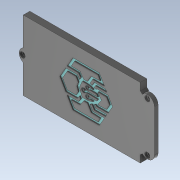
# Autodesk Inventor part: BodyBotSup
Saved by Autodesk Inventor 2020 (Build 240168000, 168)
## iProperties
Created: 2020-02-29
Part Number: BodyBotSup
Material: Generic
Document SubType Name: Modeling
Designer: Turing
Density: 1 g/cm^3
Appearance: Smooth - Black
Mass: 46.7134 g
Surface Area: 265.653 cm^2
Volume: 46.7134 cm^3
Author: Turing
Autodesk Inventor part; units mm, degrees
ref_plane "YZ Plane" through (0, 0, 0) normal (1, 0, 0) x (0, 1, 0)
ref_plane "XZ Plane" through (0, 0, 0) normal (0, 1, 0) x (-1, 0, 0)
ref_plane "XY Plane" through (0, 0, 0) normal (0, 0, 1) x (1, 0, 0)
sketch "Sketch1" plane through (0, 0, 0) normal (0, 0, 1) x (1, 0, 0)
  circle A0 centre (-91.4877, 59.6152) radius 5 projected
  circle A1 centre (0, -76.8001) radius 5 projected
  circle A2 centre (91.4877, 59.6152) radius 5 projected
  circle A3 centre (91.4877, -59.6152) radius 5 projected
  circle A4 centre (-91.4877, -59.6152) radius 5 projected
  circle A5 centre (0, 76.8001) radius 5 projected
  line L0 (-72.1, 6.8739) -> (-72.1, 37.6) projected
  line L1 (-72.1, 37.6) -> (53.9, 37.6) projected
  line L2 (53.9, 37.6) -> (53.9, 29.7386) projected
  line L3 (53.9, 29.7386) -> (56.1, 27.699) projected
  arc A6 (69.1, 22.6) -> (56.1, 27.699) centre (61.6, 22.6) ccw projected
  line L4 (69.1, 22.6) -> (69.1, -22.6) projected
  arc A7 (56.1, -27.699) -> (69.1, -22.6) centre (61.6, -22.6) ccw projected
  line L5 (56.1, -27.699) -> (53.9, -29.7386) projected
  line L6 (53.9, -29.7386) -> (53.9, -37.6) projected
  line L7 (53.9, -37.6) -> (-72.1, -37.6) projected
  line L8 (-72.1, -37.6) -> (-72.1, -6.8739) projected
  arc A8 (-72.1, 6.8739) -> (-72.1, -6.8739) centre (-69.1, 0) ccw projected
  line L9 (53.9, 29.7386) -> (56.1, 27.699) projected
  line L10 (53.9, 37.6) -> (53.9, 29.7386) projected
  line L11 (-72.1, 37.6) -> (53.9, 37.6) projected
  line L12 (-72.1, 6.8739) -> (-72.1, 37.6) projected
  arc A9 (-69.1, 7.5) -> (-72.1, 6.8739) centre (-69.1, 0) ccw projected
  line L13 (-69.1, 34.6) -> (-69.1, 7.5) projected
  line L14 (50.9, 34.6) -> (-69.1, 34.6) projected
  line L15 (50.9, 26.6) -> (50.9, 34.6) projected
  line L16 (-60, 26.6) -> (50.9, 26.6) projected
  line L17 (-60, 22.6) -> (-60, 26.6) projected
  line L18 (54.1, 22.6) -> (-60, 22.6) projected
  arc A10 (56.1, 27.699) -> (54.1, 22.6) centre (61.6, 22.6) ccw projected
  line L19 (53.9, -37.6) -> (-72.1, -37.6) projected
  line L20 (53.9, -29.7386) -> (53.9, -37.6) projected
  line L21 (56.1, -27.699) -> (53.9, -29.7386) projected
  arc A11 (54.1, -22.6) -> (56.1, -27.699) centre (61.6, -22.6) ccw projected
  line L22 (-60, -22.6) -> (54.1, -22.6) projected
  line L23 (-60, -26.6) -> (-60, -22.6) projected
  line L24 (50.9, -26.6) -> (-60, -26.6) projected
  line L25 (50.9, -34.6) -> (50.9, -26.6) projected
  line L26 (-69.1, -34.6) -> (50.9, -34.6) projected
  line L27 (-69.1, -7.5) -> (-69.1, -34.6) projected
  arc A12 (-72.1, -6.8739) -> (-69.1, -7.5) centre (-69.1, 0) ccw projected
  line L28 (-72.1, -37.6) -> (-72.1, -6.8739) projected
  circle A13 centre (-72.85, 0) radius 1.5 projected
  circle A14 centre (61.6, -26.35) radius 1.5 projected
  circle A15 centre (61.6, 26.35) radius 1.5 projected
  line L29 (-77.315, -35.1795) -> (-80.415, -33.3898) projected
  line L30 (-80.415, -33.3898) -> (-80.415, -29.8103) projected
  line L31 (-80.415, -29.8103) -> (-77.315, -28.0205) projected
  line L32 (-77.315, -28.0205) -> (-74.2151, -29.8102) projected
  line L33 (-74.2151, -29.8102) -> (-74.2151, -33.3897) projected
  line L34 (-74.2151, -33.3897) -> (-77.315, -35.1795) projected
  line L35 (-1.7898, 50.8) -> (1.7897, 50.8) projected
  line L36 (1.7897, 50.8) -> (3.5795, 47.7) projected
  line L37 (3.5795, 47.7) -> (1.7897, 44.6001) projected
  line L38 (1.7897, 44.6001) -> (-1.7898, 44.6001) projected
  line L39 (-1.7898, 44.6001) -> (-3.5795, 47.7) projected
  line L40 (-3.5795, 47.7) -> (-1.7898, 50.8) projected
  line L41 (-74.2151, 33.3898) -> (-74.2151, 29.8103) projected
  line L42 (-74.2151, 29.8103) -> (-77.315, 28.0205) projected
  line L43 (-77.315, 28.0205) -> (-80.415, 29.8102) projected
  line L44 (-80.415, 29.8102) -> (-80.415, 33.3897) projected
  line L45 (-80.415, 33.3897) -> (-77.315, 35.1795) projected
  line L46 (-77.315, 35.1795) -> (-74.2151, 33.3898) projected
  line L47 (1.7897, -50.8) -> (-1.7898, -50.8) projected
  line L48 (-1.7898, -50.8) -> (-3.5795, -47.7) projected
  line L49 (-3.5795, -47.7) -> (-1.7898, -44.6001) projected
  line L50 (-1.7898, -44.6001) -> (1.7897, -44.6001) projected
  line L51 (1.7897, -44.6001) -> (3.5795, -47.7) projected
  line L52 (3.5795, -47.7) -> (1.7897, -50.8) projected
  line L53 (94.3529, -43.81) -> (76.3482, 0) projected
  line L54 (76.3482, 0) -> (94.3529, 43.81) projected
  arc A16 (13.202, 67.65) -> (75.5922, 62.4195) centre (47.6542, 103.886) ccw projected
  line L55 (13.202, 67.65) -> (13.202, 85.3001) projected
  line L56 (-13.202, 85.3001) -> (-13.202, 67.65) projected
  arc A17 (-75.5922, 62.4195) -> (-13.202, 67.65) centre (-47.6542, 103.886) ccw projected
  line L57 (-75.5922, 62.4195) -> (-75.6824, 62.4804) projected
  line L58 (-106.8333, 56.2904) -> (-94.3529, 43.81) projected
  arc A18 (-94.3529, -43.81) -> (-94.3529, 43.81) centre (-249.3974, 0) ccw projected
  line L59 (-94.3529, -43.81) -> (-106.8333, -56.2904) projected
  line L60 (-75.6824, -62.4804) -> (-75.5922, -62.4195) projected
  arc A19 (-13.202, -67.65) -> (-75.5922, -62.4195) centre (-47.6542, -103.886) ccw projected
  line L61 (-13.202, -67.65) -> (-13.202, -85.3001) projected
  line L62 (13.202, -85.3001) -> (13.202, -67.65) projected
  arc A20 (75.5922, -62.4195) -> (13.202, -67.65) centre (47.6542, -103.886) ccw projected
  line L63 (75.5922, -62.4195) -> (75.6824, -62.4804) projected
  line L64 (75.6824, 62.4804) -> (75.5922, 62.4195) projected
  line L65 (33.8659, -51.2632) -> (32.0761, -48.1632) projected
  line L66 (32.0761, -48.1632) -> (33.8659, -45.0632) projected
  line L67 (33.8659, -45.0632) -> (37.4454, -45.0632) projected
  line L68 (37.4454, -45.0632) -> (39.2352, -48.1632) projected
  line L69 (39.2352, -48.1632) -> (37.4454, -51.2632) projected
  line L70 (37.4454, -51.2632) -> (33.8659, -51.2632) projected
  line L71 (33.8659, 51.2632) -> (37.4454, 51.2632) projected
  line L72 (37.4454, 51.2632) -> (39.2352, 48.1632) projected
  line L73 (39.2352, 48.1632) -> (37.4454, 45.0632) projected
  line L74 (37.4454, 45.0632) -> (33.8659, 45.0632) projected
  line L75 (33.8659, 45.0632) -> (32.0761, 48.1632) projected
  line L76 (32.0761, 48.1632) -> (33.8659, 51.2632) projected
  line L77 (-37.4454, -51.2632) -> (-39.2352, -48.1632) projected
  line L78 (-39.2352, -48.1632) -> (-37.4454, -45.0632) projected
  line L79 (-37.4454, -45.0632) -> (-33.8659, -45.0632) projected
  line L80 (-33.8659, -45.0632) -> (-32.0761, -48.1632) projected
  line L81 (-32.0761, -48.1632) -> (-33.8659, -51.2632) projected
  line L82 (-33.8659, -51.2632) -> (-37.4454, -51.2632) projected
  line L83 (-33.8659, 51.2632) -> (-32.0761, 48.1632) projected
  line L84 (-32.0761, 48.1632) -> (-33.8659, 45.0632) projected
  line L85 (-33.8659, 45.0632) -> (-37.4454, 45.0632) projected
  line L86 (-37.4454, 45.0632) -> (-39.2352, 48.1632) projected
  line L87 (-39.2352, 48.1632) -> (-37.4454, 51.2632) projected
  line L88 (-37.4454, 51.2632) -> (-33.8659, 51.2632) projected
  arc A21 (13.202, 85.3001) -> (-13.202, 85.3001) centre (0, 85.3001) ccw projected
  line L89 (-75.6824, 62.4804) -> (-88.1629, 74.9609) projected
  arc A22 (-88.1629, 74.9609) -> (-106.8333, 56.2904) centre (-97.4981, 65.6256) ccw projected
  arc A23 (-106.8333, -56.2904) -> (-88.1629, -74.9609) centre (-97.4981, -65.6256) ccw projected
  line L90 (-88.1629, -74.9609) -> (-75.6824, -62.4804) projected
  arc A24 (-13.202, -85.3001) -> (13.202, -85.3001) centre (0, -85.3001) ccw projected
  line L91 (75.6824, -62.4804) -> (88.1629, -74.9609) projected
  arc A25 (88.1629, -74.9609) -> (106.8333, -56.2904) centre (97.4981, -65.6256) ccw projected
  line L92 (106.8333, -56.2904) -> (94.3529, -43.81) projected
  line L93 (94.3529, 43.81) -> (106.8333, 56.2904) projected
  arc A26 (106.8333, 56.2904) -> (88.1629, 74.9609) centre (97.4981, 65.6256) ccw projected
  line L94 (88.1629, 74.9609) -> (75.6824, 62.4804) projected
  point P0 (0, 0)
extrude "Extrusion1" add sketch "Sketch1" against normal blind 4 contours A9 L13 L14 L15 L16 L17 L18 A10 A6 L4 A7 A11 L22 L23 L24 L25 L26 L27 A12 A8
sketch "Sketch2" plane through (0, 0, 0) normal (0, 0, 1) x (1, 0, 0)
  circle A0 centre (-91.4877, 59.6152) radius 5 projected
  circle A1 centre (0, -76.8001) radius 5 projected
  circle A2 centre (91.4877, 59.6152) radius 5 projected
  circle A3 centre (91.4877, -59.6152) radius 5 projected
  circle A4 centre (-91.4877, -59.6152) radius 5 projected
  circle A5 centre (0, 76.8001) radius 5 projected
  line L0 (-72.1, 6.8739) -> (-72.1, 37.6) projected
  line L1 (-72.1, 37.6) -> (53.9, 37.6) projected
  line L2 (53.9, 37.6) -> (53.9, 29.7386) projected
  line L3 (53.9, 29.7386) -> (56.1, 27.699) projected
  arc A6 (69.1, 22.6) -> (56.1, 27.699) centre (61.6, 22.6) ccw projected
  line L4 (69.1, 22.6) -> (69.1, -22.6) projected
  arc A7 (56.1, -27.699) -> (69.1, -22.6) centre (61.6, -22.6) ccw projected
  line L5 (56.1, -27.699) -> (53.9, -29.7386) projected
  line L6 (53.9, -29.7386) -> (53.9, -37.6) projected
  line L7 (53.9, -37.6) -> (-72.1, -37.6) projected
  line L8 (-72.1, -37.6) -> (-72.1, -6.8739) projected
  arc A8 (-72.1, 6.8739) -> (-72.1, -6.8739) centre (-69.1, 0) ccw projected
  line L9 (53.9, 29.7386) -> (56.1, 27.699) projected
  line L10 (53.9, 37.6) -> (53.9, 29.7386) projected
  line L11 (-72.1, 37.6) -> (53.9, 37.6) projected
  line L12 (-72.1, 6.8739) -> (-72.1, 37.6) projected
  arc A9 (-69.1, 7.5) -> (-72.1, 6.8739) centre (-69.1, 0) ccw projected
  line L13 (-69.1, 34.6) -> (-69.1, 7.5) projected
  line L14 (50.9, 34.6) -> (-69.1, 34.6) projected
  line L15 (50.9, 26.6) -> (50.9, 34.6) projected
  line L16 (-60, 26.6) -> (50.9, 26.6) projected
  line L17 (-60, 22.6) -> (-60, 26.6) projected
  line L18 (54.1, 22.6) -> (-60, 22.6) projected
  arc A10 (56.1, 27.699) -> (54.1, 22.6) centre (61.6, 22.6) ccw projected
  line L19 (53.9, -37.6) -> (-72.1, -37.6) projected
  line L20 (53.9, -29.7386) -> (53.9, -37.6) projected
  line L21 (56.1, -27.699) -> (53.9, -29.7386) projected
  arc A11 (54.1, -22.6) -> (56.1, -27.699) centre (61.6, -22.6) ccw projected
  line L22 (-60, -22.6) -> (54.1, -22.6) projected
  line L23 (-60, -26.6) -> (-60, -22.6) projected
  line L24 (50.9, -26.6) -> (-60, -26.6) projected
  line L25 (50.9, -34.6) -> (50.9, -26.6) projected
  line L26 (-69.1, -34.6) -> (50.9, -34.6) projected
  line L27 (-69.1, -7.5) -> (-69.1, -34.6) projected
  arc A12 (-72.1, -6.8739) -> (-69.1, -7.5) centre (-69.1, 0) ccw projected
  line L28 (-72.1, -37.6) -> (-72.1, -6.8739) projected
  line L29 (-77.315, -35.1795) -> (-80.415, -33.3898) projected
  line L30 (-80.415, -33.3898) -> (-80.415, -29.8103) projected
  line L31 (-80.415, -29.8103) -> (-77.315, -28.0205) projected
  line L32 (-77.315, -28.0205) -> (-74.2151, -29.8102) projected
  line L33 (-74.2151, -29.8102) -> (-74.2151, -33.3897) projected
  line L34 (-74.2151, -33.3897) -> (-77.315, -35.1795) projected
  line L35 (-1.7898, 50.8) -> (1.7897, 50.8) projected
  line L36 (1.7897, 50.8) -> (3.5795, 47.7) projected
  line L37 (3.5795, 47.7) -> (1.7897, 44.6001) projected
  line L38 (1.7897, 44.6001) -> (-1.7898, 44.6001) projected
  line L39 (-1.7898, 44.6001) -> (-3.5795, 47.7) projected
  line L40 (-3.5795, 47.7) -> (-1.7898, 50.8) projected
  line L41 (-74.2151, 33.3898) -> (-74.2151, 29.8103) projected
  line L42 (-74.2151, 29.8103) -> (-77.315, 28.0205) projected
  line L43 (-77.315, 28.0205) -> (-80.415, 29.8102) projected
  line L44 (-80.415, 29.8102) -> (-80.415, 33.3897) projected
  line L45 (-80.415, 33.3897) -> (-77.315, 35.1795) projected
  line L46 (-77.315, 35.1795) -> (-74.2151, 33.3898) projected
  line L47 (1.7897, -50.8) -> (-1.7898, -50.8) projected
  line L48 (-1.7898, -50.8) -> (-3.5795, -47.7) projected
  line L49 (-3.5795, -47.7) -> (-1.7898, -44.6001) projected
  line L50 (-1.7898, -44.6001) -> (1.7897, -44.6001) projected
  line L51 (1.7897, -44.6001) -> (3.5795, -47.7) projected
  line L52 (3.5795, -47.7) -> (1.7897, -50.8) projected
  line L53 (94.3529, -43.81) -> (76.3482, 0) projected
  line L54 (76.3482, 0) -> (94.3529, 43.81) projected
  arc A13 (13.202, 67.65) -> (75.5922, 62.4195) centre (47.6542, 103.886) ccw projected
  line L55 (13.202, 67.65) -> (13.202, 85.3001) projected
  line L56 (-13.202, 85.3001) -> (-13.202, 67.65) projected
  arc A14 (-75.5922, 62.4195) -> (-13.202, 67.65) centre (-47.6542, 103.886) ccw projected
  line L57 (-75.5922, 62.4195) -> (-75.6824, 62.4804) projected
  line L58 (-106.8333, 56.2904) -> (-94.3529, 43.81) projected
  arc A15 (-94.3529, -43.81) -> (-94.3529, 43.81) centre (-249.3974, 0) ccw projected
  line L59 (-94.3529, -43.81) -> (-106.8333, -56.2904) projected
  line L60 (-75.6824, -62.4804) -> (-75.5922, -62.4195) projected
  arc A16 (-13.202, -67.65) -> (-75.5922, -62.4195) centre (-47.6542, -103.886) ccw projected
  line L61 (-13.202, -67.65) -> (-13.202, -85.3001) projected
  line L62 (13.202, -85.3001) -> (13.202, -67.65) projected
  arc A17 (75.5922, -62.4195) -> (13.202, -67.65) centre (47.6542, -103.886) ccw projected
  line L63 (75.5922, -62.4195) -> (75.6824, -62.4804) projected
  line L64 (75.6824, 62.4804) -> (75.5922, 62.4195) projected
  line L65 (33.8659, -51.2632) -> (32.0761, -48.1632) projected
  line L66 (32.0761, -48.1632) -> (33.8659, -45.0632) projected
  line L67 (33.8659, -45.0632) -> (37.4454, -45.0632) projected
  line L68 (37.4454, -45.0632) -> (39.2352, -48.1632) projected
  line L69 (39.2352, -48.1632) -> (37.4454, -51.2632) projected
  line L70 (37.4454, -51.2632) -> (33.8659, -51.2632) projected
  line L71 (33.8659, 51.2632) -> (37.4454, 51.2632) projected
  line L72 (37.4454, 51.2632) -> (39.2352, 48.1632) projected
  line L73 (39.2352, 48.1632) -> (37.4454, 45.0632) projected
  line L74 (37.4454, 45.0632) -> (33.8659, 45.0632) projected
  line L75 (33.8659, 45.0632) -> (32.0761, 48.1632) projected
  line L76 (32.0761, 48.1632) -> (33.8659, 51.2632) projected
  line L77 (-37.4454, -51.2632) -> (-39.2352, -48.1632) projected
  line L78 (-39.2352, -48.1632) -> (-37.4454, -45.0632) projected
  line L79 (-37.4454, -45.0632) -> (-33.8659, -45.0632) projected
  line L80 (-33.8659, -45.0632) -> (-32.0761, -48.1632) projected
  line L81 (-32.0761, -48.1632) -> (-33.8659, -51.2632) projected
  line L82 (-33.8659, -51.2632) -> (-37.4454, -51.2632) projected
  line L83 (-33.8659, 51.2632) -> (-32.0761, 48.1632) projected
  line L84 (-32.0761, 48.1632) -> (-33.8659, 45.0632) projected
  line L85 (-33.8659, 45.0632) -> (-37.4454, 45.0632) projected
  line L86 (-37.4454, 45.0632) -> (-39.2352, 48.1632) projected
  line L87 (-39.2352, 48.1632) -> (-37.4454, 51.2632) projected
  line L88 (-37.4454, 51.2632) -> (-33.8659, 51.2632) projected
  arc A18 (13.202, 85.3001) -> (-13.202, 85.3001) centre (0, 85.3001) ccw projected
  line L89 (-75.6824, 62.4804) -> (-88.1629, 74.9609) projected
  arc A19 (-88.1629, 74.9609) -> (-106.8333, 56.2904) centre (-97.4981, 65.6256) ccw projected
  arc A20 (-106.8333, -56.2904) -> (-88.1629, -74.9609) centre (-97.4981, -65.6256) ccw projected
  line L90 (-88.1629, -74.9609) -> (-75.6824, -62.4804) projected
  arc A21 (-13.202, -85.3001) -> (13.202, -85.3001) centre (0, -85.3001) ccw projected
  line L91 (75.6824, -62.4804) -> (88.1629, -74.9609) projected
  arc A22 (88.1629, -74.9609) -> (106.8333, -56.2904) centre (97.4981, -65.6256) ccw projected
  line L92 (106.8333, -56.2904) -> (94.3529, -43.81) projected
  line L93 (94.3529, 43.81) -> (106.8333, 56.2904) projected
  arc A23 (106.8333, 56.2904) -> (88.1629, 74.9609) centre (97.4981, 65.6256) ccw projected
  line L94 (88.1629, 74.9609) -> (75.6824, 62.4804) projected
  point P0 (0, 0)
extrude "Extrusion2" add sketch "Sketch2" against normal blind 7 contours L0 L1 L2 L3 A10 L18 L17 L16 L15 L14 L13 A9 | A12 L27 L26 L25 L24 L23 L22 A11 L5 L6 L7 L8
sketch "Sketch3" plane through (0, 0, 0) normal (0, 0, 1) x (1, 0, 0)
  line L0 (-72.1, -6.8739) -> (-72.1, -37.6) projected
  line L1 (-72.1, -37.6) -> (53.9, -37.6) projected
  line L2 (53.9, -37.6) -> (53.9, -29.7386) projected
  line L3 (53.9, -29.7386) -> (56.1, -27.699) projected
  arc A0 (56.1, -27.699) -> (69.1, -22.6) centre (61.6, -22.6) ccw projected
  line L4 (69.1, -22.6) -> (69.1, 22.6) projected
  arc A1 (69.1, 22.6) -> (56.1, 27.699) centre (61.6, 22.6) ccw projected
  line L5 (56.1, 27.699) -> (53.9, 29.7386) projected
  line L6 (53.9, 29.7386) -> (53.9, 37.6) projected
  line L7 (53.9, 37.6) -> (-72.1, 37.6) projected
  line L8 (-72.1, 37.6) -> (-72.1, 6.8739) projected
  arc A2 (-72.1, 6.8739) -> (-72.1, -6.8739) centre (-69.1, 0) ccw projected
  circle A3 centre (61.6, 26.35) radius 1.5 projected
  circle A4 centre (-72.85, 0) radius 1.5 projected
  circle A5 centre (61.6, -26.35) radius 1.5 projected
  circle A6 centre (61.6, -26.35) radius 2.8
  circle A7 centre (61.6, 26.35) radius 2.8
  circle A8 centre (-72.85, 0) radius 2.8
  point P0 (0, 0)
  dimension "d4" = 5.6
  dimension "d5" = 5.6
  dimension "d6" = 5.6
  constraints: 3 centre point, 3 coincident
  measures "d4" diameter of A6
  measures "d5" diameter of A7
  measures "d6" diameter of A8
extrude "Extrusion3" cut sketch "Sketch3" against normal blind 2 contours A3 | A4 | A5 | A6 | A7 | A8
sketch "Sketch6" plane through (0, 0, 0) normal (0, 0, 1) x (1, 0, 0)
  line L0 (9.8592, -24.4421) -> (15.3959, -14.8899)
  line L1 (15.3959, -14.8899) -> (2.6739, -14.8899)
  line L2 (2.6739, -14.8899) -> (-0.2047, -9.9039)
  line L3 (-0.2047, -9.9039) -> (1.9763, -8.9847)
  line L4 (1.9763, -8.9847) -> (4.2927, -12.9968)
  line L5 (4.2927, -12.9968) -> (16.6236, -12.7718)
  line L6 (16.6236, -12.7718) -> (17.854, -10.4095)
  line L7 (17.854, -10.4095) -> (5.6643, -10.4095)
  line L8 (5.6643, -10.4095) -> (4.2809, -8.0134)
  line L9 (4.2809, -8.0134) -> (6.1857, -7.2106)
  line L10 (6.1857, -7.2106) -> (6.9752, -8.3147)
  line L11 (6.9752, -8.3147) -> (19.2071, -8.3147)
  line L12 (19.2071, -8.3147) -> (24.0266, 0)
  line L13 (24.0266, 0) -> (19.2071, 8.3147)
  line L14 (19.2071, 8.3147) -> (6.9752, 8.3147)
  line L15 (6.9752, 8.3147) -> (6.1857, 7.2106)
  line L16 (6.1857, 7.2106) -> (4.2809, 8.0134)
  line L17 (4.2809, 8.0134) -> (5.6643, 10.4095)
  line L18 (5.6643, 10.4095) -> (17.854, 10.4095)
  line L19 (17.854, 10.4095) -> (16.6236, 12.7718)
  line L20 (16.6236, 12.7718) -> (4.2927, 12.9968)
  line L21 (4.2927, 12.9968) -> (1.9763, 8.9847)
  line L22 (1.9763, 8.9847) -> (-0.2047, 9.9039)
  line L23 (-0.2047, 9.9039) -> (2.6739, 14.8899)
  line L24 (2.6739, 14.8899) -> (15.3959, 14.8899)
  line L25 (15.3959, 14.8899) -> (9.8592, 24.4421)
  line L26 (9.8592, 24.4421) -> (-18.6408, 24.4421)
  line L27 (-18.6408, 24.4421) -> (-24.9408, 13.5301)
  line L28 (-24.9408, 13.5301) -> (-12.5648, 13.3043)
  line L29 (-12.5648, 13.3043) -> (-10.378, 10.186)
  line L30 (-10.378, 10.186) -> (-11.5351, 7.7835)
  line L31 (-11.5351, 7.7835) -> (-13.8681, 11.1103)
  line L32 (-13.8681, 11.1103) -> (-26.3379, 11.1103)
  line L33 (-26.3379, 11.1103) -> (-32.7525, 0)
  line L34 (-32.7525, 0) -> (-26.3379, -11.1103)
  line L35 (-26.3379, -11.1103) -> (-13.8681, -11.1103)
  line L36 (-13.8681, -11.1103) -> (-11.5351, -7.7835)
  line L37 (-11.5351, -7.7835) -> (-10.378, -10.186)
  line L38 (-10.378, -10.186) -> (-12.5648, -13.3043)
  line L39 (-12.5648, -13.3043) -> (-24.9408, -13.5301)
  line L40 (-24.9408, -13.5301) -> (-18.6408, -24.4421)
  line L41 (-18.6408, -24.4421) -> (9.8592, -24.4421)
  line L42 (-24.8186, -8.6442) -> (-29.8221, 0)
  line L43 (-29.8221, 0) -> (-24.8186, 8.6442)
  line L44 (-24.8186, 8.6442) -> (-15.3299, 8.6442)
  line L45 (-15.3299, 8.6442) -> (-13.2333, 5)
  line L46 (-13.2333, 5) -> (-12.9845, 4.1573)
  line L47 (-12.9845, 4.1573) -> (-14.4186, 0)
  line L48 (-14.4186, 0) -> (-12.9845, -4.1573)
  line L49 (-12.9845, -4.1573) -> (-13.2333, -5)
  line L50 (-13.2333, -5) -> (-15.3299, -8.6442)
  line L51 (-15.3299, -8.6442) -> (-24.8186, -8.6442)
  spline S0 degree 4 poles (2.9355, 5.8382) (3.2225, 5.7092) (3.4051, 5.5552) (3.4376, 5.5163) (3.429, 5.4648) (3.396, 5.4265) (3.0418, 5.3486) (1.972, 5.2666) (0.3846, 5.208) (-0.4495, 5.2778) (-0.7892, 5.3625) (-1.3167, 5.6157) (-1.7386, 5.9196) (-2.1891, 6.197) (-2.7133, 6.3284) (-3.1987, 6.3284) (-3.6089, 6.2229) (-4.1539, 5.9196) (-4.5249, 5.5551) (-4.7492, 5.2414) (-4.9527, 4.7585) (-5.0176, 4.6444) (-5.0176, 4.1047) (-4.9305, 3.6022) (-4.6213, 3.0688) (-4.4627, 2.8378) (-4.1539, 2.5446) (-3.6529, 2.2543) (-3.1738, 2.1638) (-2.7133, 2.1638) (-2.2752, 2.2683) (-1.8947, 2.4397) (-1.5879, 2.6714) (-1.2968, 2.9582) (-1.0715, 3.1097) (-0.657, 3.1924) (-0.2047, 3.2593) (0.4426, 3.291) (1.1568, 3.291) (2.0681, 3.291) (6.7773, 3.291) knots 1 1 1 1 1 2 3 4 5 6 7 8 9 10 11 12 13 14 15 16 17 18 19 20 21 22 23 24 25 26 27 28 29 30 31 32 33 34 35 36 37 38 38 38 38 38
  spline S1 degree 4 poles (6.7773, 3.291) (8.1865, 1.3872) (8.2483, 1.1897) (8.245, 1.1839) (8.235, 1.1666) (8.2078, 1.1586) (7.997, 1.1586) (6.1055, 1.066) (4.4293, 1.066) (2.1767, 1.0161) (-0.527, 1.016) (-2.6244, 1.016) (-3.4141, 1.1017) (-4.2327, 1.1771) (-4.6821, 1.4365) (-4.9023, 1.5605) (-5.5001, 1.8854) (-6.3079, 2.3096) (-6.586, 2.379) (-7.2919, 2.3444) (-7.8873, 2.1537) (-8.3696, 1.8741) (-8.671, 1.5628) (-8.9681, 1.2948) (-9.1907, 0.8325) (-9.2113, 0.7969) (-9.2612, 0.5978) (-9.2986, 0.3588) (-9.2986, 0.1317) (-9.2986, 0) knots 1 1 1 1 1 2 3 4 5 6 7 8 9 10 11 12 13 14 15 16 17 18 19 20 21 22 23 24 25 26 27 27 27 27 27
  spline S2 degree 4 poles (-9.2986, 0) (-9.2986, -0.1318) (-9.2986, -0.3588) (-9.2612, -0.5978) (-9.2113, -0.7969) (-9.1907, -0.8325) (-8.9681, -1.2948) (-8.671, -1.5628) (-8.3696, -1.8742) (-7.8873, -2.1537) (-7.2919, -2.3444) (-6.586, -2.379) (-6.3079, -2.3096) (-5.5001, -1.8855) (-4.9023, -1.5605) (-4.6821, -1.4365) (-4.2327, -1.1771) (-3.4141, -1.1017) (-2.6244, -1.0161) (-0.527, -1.016) (2.1767, -1.016) (4.4293, -1.066) (6.1055, -1.066) (7.997, -1.1585) (8.2078, -1.1585) (8.235, -1.1666) (8.245, -1.1839) (8.2483, -1.1896) (8.1865, -1.3872) (6.7773, -3.291) knots 1 1 1 1 1 2 3 4 5 6 7 8 9 10 11 12 13 14 15 16 17 18 19 20 21 22 23 24 25 26 27 27 27 27 27
  spline S3 degree 4 poles (6.7773, -3.291) (2.0681, -3.291) (1.1568, -3.291) (0.4426, -3.291) (-0.2047, -3.2593) (-0.657, -3.1924) (-1.0715, -3.1097) (-1.2968, -2.9582) (-1.5879, -2.6714) (-1.8947, -2.4397) (-2.2752, -2.2683) (-2.7133, -2.1638) (-3.1738, -2.1638) (-3.6529, -2.2543) (-4.1539, -2.5447) (-4.4627, -2.8379) (-4.6213, -3.0688) (-4.9305, -3.6022) (-5.0176, -4.1047) (-5.0176, -4.6444) (-4.9527, -4.7586) (-4.7492, -5.2414) (-4.5249, -5.5552) (-4.1539, -5.9196) (-3.6089, -6.223) (-3.1987, -6.3285) (-2.7133, -6.3285) (-2.1891, -6.1971) (-1.7386, -5.9196) (-1.3167, -5.6157) (-0.7892, -5.3625) (-0.4495, -5.2778) (0.3846, -5.208) (1.972, -5.2666) (3.0418, -5.3486) (3.396, -5.4265) (3.429, -5.4648) (3.4376, -5.5163) (3.4051, -5.5552) (3.2225, -5.7092) (2.9355, -5.8382) knots 1 1 1 1 1 2 3 4 5 6 7 8 9 10 11 12 13 14 15 16 17 18 19 20 21 22 23 24 25 26 27 28 29 30 31 32 33 34 35 36 37 38 38 38 38 38
  spline S4 degree 4 poles (2.9355, -5.8382) (2.4814, -6.1119) (-0.0379, -6.9283) (-1.1698, -7.2106) (-2.7133, -7.3528) (-5.5946, -7.5458) (-7.4089, -7.457) (-8.4358, -7.457) (-8.7669, -7.265) (-8.9681, -6.5471) (-9.6744, -4.8713) (-10.531, -2.9004) (-10.9566, -1.719) (-11.2264, -0.8707) (-11.3924, -0.2455) (-11.3924, 0) knots 1 1 1 1 1 2 3 4 5 6 7 8 9 10 11 12 13 13 13 13 13
  spline S5 degree 4 poles (-11.3924, 0) (-11.3924, 0.2455) (-11.2264, 0.8707) (-10.9566, 1.7189) (-10.531, 2.9003) (-9.6744, 4.8713) (-8.9681, 6.5471) (-8.767, 7.265) (-8.4359, 7.4569) (-7.4089, 7.4569) (-5.5946, 7.5457) (-2.7133, 7.3528) (-1.1698, 7.2106) (-0.0379, 6.9284) (2.4814, 6.1119) (2.9355, 5.8382) knots 1 1 1 1 1 2 3 4 5 6 7 8 9 10 11 12 13 13 13 13 13
  line L52 (10.7244, 17.5129) -> (1.0307, 17.0384)
  line L53 (1.0307, 17.0384) -> (-3.1738, 10.1143)
  line L54 (-3.1738, 10.1143) -> (-7.1007, 10.186)
  line L55 (-7.1007, 10.186) -> (-10.9566, 15.6436)
  line L56 (-10.9566, 15.6436) -> (-20.4829, 15.8176)
  line L57 (-20.4829, 15.8176) -> (-16.9796, 21.8855)
  line L58 (-16.9796, 21.8855) -> (8.374, 21.8855)
  line L59 (8.374, 21.8855) -> (10.7244, 17.5129)
  line L60 (17.4812, 5.8382) -> (20.8652, 0)
  line L61 (20.8652, 0) -> (17.4812, -5.8382)
  line L62 (17.4812, -5.8382) -> (8.5584, -6.001)
  line L63 (8.5584, -6.001) -> (8.2855, -5.5552)
  line L64 (8.2855, -5.5552) -> (12.0089, -0.2455)
  line L65 (12.0089, -0.2455) -> (12.0089, 0.2455)
  line L66 (12.0089, 0.2455) -> (8.2855, 5.5552)
  line L67 (8.2855, 5.5552) -> (8.5584, 6.001)
  line L68 (8.5584, 6.001) -> (17.4812, 5.8382)
  line L69 (-7.1007, -10.186) -> (-3.1738, -10.1143)
  line L70 (-3.1738, -10.1143) -> (1.0307, -17.0384)
  line L71 (1.0307, -17.0384) -> (10.7244, -17.5129)
  line L72 (10.7244, -17.5129) -> (8.374, -21.8855)
  line L73 (8.374, -21.8855) -> (-16.9796, -21.8855)
  line L74 (-16.9796, -21.8855) -> (-20.4829, -15.8176)
  line L75 (-20.4829, -15.8176) -> (-10.9566, -15.6436)
  line L76 (-10.9566, -15.6436) -> (-7.1007, -10.186)
  line L77 (53.9, 37.6) -> (-72.1, 37.6) projected
  circle A0 centre (-2.9578, -4.3221) radius 1.0532
  circle A1 centre (-7.2867, 0) radius 1.1853
  circle A2 centre (-3.1738, 4.1262) radius 1.0241
  point P0 (0, 0)
  point P1 (-5.9112, 0)
  constraints: 154 end point, 3 centre point, 12 other
extrude "Extrusion5" cut sketch "Sketch6" against normal blind 1
equation "\"d5\" = d4"
equation "\"d6\" = d4"
body "Solid1"
